Autodesk Inventor part; units mm, degrees
(part 3 of 7)
  line L373 (-46.0236, -59.4146) -> (-46.4209, -59.4428)
  line L374 (-46.4209, -59.4428) -> (-47.351, -59.469)
  line L375 (-47.351, -59.469) -> (-48.2632, -59.4537)
  line L376 (-48.2632, -59.4537) -> (-48.6381, -59.4301)
  line L377 (-48.6381, -59.4301) -> (-48.9193, -59.3956)
  line L378 (-48.9193, -59.3956) -> (-49.5759, -59.2467)
  line L379 (-49.5759, -59.2467) -> (-49.8747, -59.1544)
  line L380 (-49.8747, -59.1544) -> (-50.1547, -59.0499)
  line L381 (-50.1547, -59.0499) -> (-50.4164, -58.9329)
  line L382 (-50.4164, -58.9329) -> (-50.6606, -58.8031)
  line L383 (-50.6606, -58.8031) -> (-50.8877, -58.6602)
  line L384 (-50.8877, -58.6602) -> (-51.0986, -58.5041)
  line L385 (-51.0986, -58.5041) -> (-51.2624, -58.3746)
  line L386 (-51.2624, -58.3746) -> (-51.2624, -58.5384)
  line L387 (-51.2624, -58.5384) -> (-51.2496, -58.7821)
  line L388 (-51.2496, -58.7821) -> (-51.2138, -59.0766)
  line L389 (-51.2138, -59.0766) -> (-51.091, -59.7004)
  line L390 (-51.091, -59.7004) -> (-51.0286, -59.9871)
  line L391 (-51.0286, -59.9871) -> (-51.024, -60.0626)
  line L392 (-51.024, -60.0626) -> (-51.0376, -60.0967)
  line L393 (-51.0376, -60.0967) -> (-51.1136, -60.1071)
  line L394 (-51.1136, -60.1071) -> (-51.2372, -60.0829)
  line L395 (-51.2372, -60.0829) -> (-51.3971, -60.0265)
  line L396 (-51.3971, -60.0265) -> (-51.5825, -59.9405)
  line L397 (-51.5825, -59.9405) -> (-51.8754, -59.7765)
  line L398 (-51.8754, -59.7765) -> (-52.1087, -59.6085)
  line L399 (-52.1087, -59.6085) -> (-52.317, -59.4084)
  line L400 (-52.317, -59.4084) -> (-52.535, -59.148)
  line L401 (-52.535, -59.148) -> (-52.8359, -58.7594)
  line L402 (-52.8359, -58.7594) -> (-52.9541, -58.8318)
  line L403 (-52.9541, -58.8318) -> (-53.2253, -58.9829)
  line L404 (-53.2253, -58.9829) -> (-53.5098, -59.1066)
  line L405 (-53.5098, -59.1066) -> (-53.8365, -59.2138)
  line L406 (-53.8365, -59.2138) -> (-54.2342, -59.3156)
  line L407 (-54.2342, -59.3156) -> (-54.5443, -59.3742)
  line L408 (-54.5443, -59.3742) -> (-54.6227, -59.3762)
  line L409 (-54.6227, -59.3762) -> (-54.6571, -59.3614)
  line L410 (-54.6571, -59.3614) -> (-54.7009, -59.1688)
  line L411 (-54.7009, -59.1688) -> (-54.7357, -58.8151)
  line L412 (-54.7357, -58.8151) -> (-54.7541, -58.4136)
  line L413 (-54.7541, -58.4136) -> (-54.7486, -58.0774)
  line L414 (-54.7486, -58.0774) -> (-54.7195, -57.6626)
  line L415 (-54.7195, -57.6626) -> (-54.7329, -57.3906)
  line L416 (-54.7329, -57.3906) -> (-54.8113, -57.1344)
  line L417 (-54.8113, -57.1344) -> (-54.9772, -56.7667)
  line L418 (-54.9772, -56.7667) -> (-55.2401, -56.2067)
  line L419 (-55.2401, -56.2067) -> (-55.3772, -56.2067)
  line L420 (-55.3772, -56.2067) -> (-55.5187, -56.1843)
  line L421 (-55.5187, -56.1843) -> (-55.6744, -56.1305)
  line L422 (-55.6744, -56.1305) -> (-55.8426, -56.0168)
  line L423 (-55.8426, -56.0168) -> (-56.0768, -55.8128)
  line L424 (-56.0768, -55.8128) -> (-56.3318, -55.5609)
  line L425 (-56.3318, -55.5609) -> (-56.5621, -55.3037)
  line L426 (-56.5621, -55.3037) -> (-56.6955, -55.1437)
  line L427 (-56.6955, -55.1437) -> (-56.8631, -55.2999)
  line L428 (-56.8631, -55.2999) -> (-57.2147, -55.6065)
  line L429 (-57.2147, -55.6065) -> (-57.4899, -55.8214)
  line L430 (-57.4899, -55.8214) -> (-57.685, -55.9412)
  line L431 (-57.685, -55.9412) -> (-57.7515, -55.9645)
  line L432 (-57.7515, -55.9645) -> (-57.7966, -55.9628)
  line L433 (-57.7966, -55.9628) -> (-57.8301, -55.9383)
  line L434 (-57.8301, -55.9383) -> (-57.859, -55.8916)
  line L435 (-57.859, -55.8916) -> (-57.9018, -55.739)
  line L436 (-57.9018, -55.739) -> (-57.9225, -55.5192)
  line L437 (-57.9225, -55.5192) -> (-57.9185, -55.2466)
  line L438 (-57.9185, -55.2466) -> (-57.8994, -54.8808)
  line L439 (-57.8994, -54.8808) -> (-58.1128, -54.976)
  line L440 (-58.1128, -54.976) -> (-58.4276, -55.0851)
  line L441 (-58.4276, -55.0851) -> (-58.8824, -55.2199)
  line L442 (-58.8824, -55.2199) -> (-59.4996, -55.3913)
  line L443 (-59.4996, -55.3913) -> (-59.5345, -55.3951)
  line L444 (-59.5345, -55.3951) -> (-59.5554, -55.3789)
  line L445 (-59.5554, -55.3789) -> (-59.5682, -55.258)
  line L446 (-59.5682, -55.258) -> (-59.5539, -55.1342)
  line L447 (-59.5539, -55.1342) -> (-59.5329, -55.109)
  line L448 (-59.5329, -55.109) -> (-59.4996, -55.1018)
  line L449 (-59.4996, -55.1018) -> (-59.2636, -55.053)
  line L450 (-59.2636, -55.053) -> (-58.8515, -54.937)
  line L451 (-58.8515, -54.937) -> (-58.4158, -54.7996)
  line L452 (-58.4158, -54.7996) -> (-58.109, -54.6865)
  line L453 (-58.109, -54.6865) -> (-57.8376, -54.5834)
  line L454 (-57.8376, -54.5834) -> (-57.7515, -54.5766)
  line L455 (-57.7515, -54.5766) -> (-57.6927, -54.605)
  line L456 (-57.6927, -54.605) -> (-57.6572, -54.673)
  line L457 (-57.6572, -54.673) -> (-57.6407, -54.7845)
  line L458 (-57.6407, -54.7845) -> (-57.648, -55.1551)
  line L459 (-57.648, -55.1551) -> (-57.6585, -55.479)
  line L460 (-57.6585, -55.479) -> (-57.6404, -55.5971)
  line L461 (-57.6404, -55.5971) -> (-57.5546, -55.5456)
  line L462 (-57.5546, -55.5456) -> (-57.3856, -55.4085)
  line L463 (-57.3856, -55.4085) -> (-56.9165, -54.9799)
  line L464 (-56.9165, -54.9799) -> (-56.6841, -54.7551)
  line L465 (-56.6841, -54.7551) -> (-56.444, -55.0332)
  line L466 (-56.444, -55.0332) -> (-55.9573, -55.5656)
  line L467 (-55.9573, -55.5656) -> (-55.7882, -55.7233)
  line L468 (-55.7882, -55.7233) -> (-55.6477, -55.8295)
  line L469 (-55.6477, -55.8295) -> (-55.514, -55.9035)
  line L470 (-55.514, -55.9035) -> (-55.4153, -55.9362)
  line L471 (-55.4153, -55.9362) -> (-55.3595, -55.9259)
  line L472 (-55.3595, -55.9259) -> (-55.3544, -55.8714)
  line L473 (-55.3544, -55.8714) -> (-55.4462, -55.5283)
  line L474 (-55.4462, -55.5283) -> (-55.5234, -55.1751)
  line L475 (-55.5234, -55.1751) -> (-55.6439, -54.3817)
  line L476 (-55.6439, -54.3817) -> (-55.6632, -54.1753)
  line L477 (-55.6632, -54.1753) -> (-55.6525, -54.0593)
  line L478 (-55.6525, -54.0593) -> (-55.6332, -54.0272)
  line L479 (-55.6332, -54.0272) -> (-55.6032, -54.0082)
  line L480 (-55.6032, -54.0082) -> (-55.5068, -53.9969)
  line L481 (-55.5068, -53.9969) -> (-55.4609, -54.0075)
  line L482 (-55.4609, -54.0075) -> (-55.431, -54.0559)
  line L483 (-55.431, -54.0559) -> (-55.381, -54.3664)
  line L484 (-55.381, -54.3664) -> (-55.2779, -55.0469)
  line L485 (-55.2779, -55.0469) -> (-55.142, -55.6209)
  line L486 (-55.142, -55.6209) -> (-54.9417, -56.1935)
  line L487 (-54.9417, -56.1935) -> (-54.6457, -56.8696)
  line L488 (-54.6457, -56.8696) -> (-54.5187, -57.1502)
  line L489 (-54.5187, -57.1502) -> (-54.4528, -57.3254)
  line L490 (-54.4528, -57.3254) -> (-54.4319, -57.4499)
  line L491 (-54.4319, -57.4499) -> (-54.44, -57.5783)
  line L492 (-54.44, -57.5783) -> (-54.4923, -58.2436)
  line L493 (-54.4923, -58.2436) -> (-54.4819, -58.7403)
  line L494 (-54.4819, -58.7403) -> (-54.4552, -59.0718)
  line L495 (-54.4552, -59.0718) -> (-54.2723, -59.0489)
  line L496 (-54.2723, -59.0489) -> (-54.006, -58.9912)
  line L497 (-54.006, -58.9912) -> (-53.6994, -58.8899)
  line L498 (-53.6994, -58.8899) -> (-53.3877, -58.7585)
  line L499 (-53.3877, -58.7585) -> (-53.1065, -58.6108)
  line L500 (-53.1065, -58.6108) -> (-52.7674, -58.4165)
  line L501 (-52.7674, -58.4165) -> (-52.5197, -58.7441)
  line L502 (-52.5197, -58.7441) -> (-52.2934, -59.0362)
  line L503 (-52.2934, -59.0362) -> (-52.0778, -59.2718)
  line L504 (-52.0778, -59.2718) -> (-51.865, -59.4589)
  line L505 (-51.865, -59.4589) -> (-51.6472, -59.6052)
  line L506 (-51.6472, -59.6052) -> (-51.3881, -59.7347)
  line L507 (-51.3881, -59.7347) -> (-51.4339, -59.3842)
  line L508 (-51.4339, -59.3842) -> (-51.4843, -58.9908)
  line L509 (-51.4843, -58.9908) -> (-51.5177, -58.5232)
  line L510 (-51.5177, -58.5232) -> (-51.5258, -58.0845)
  line L511 (-51.5258, -58.0845) -> (-51.5107, -58.0051)
  line L512 (-51.5107, -58.0051) -> (-51.4796, -57.9745)
  line L513 (-51.4796, -57.9745) -> (-51.4248, -57.9843)
  line L514 (-51.4248, -57.9843) -> (-51.3243, -58.0355)
  line L515 (-51.3243, -58.0355) -> (-50.9919, -58.2565)
  line L516 (-50.9919, -58.2565) -> (-50.6288, -58.4993)
  line L517 (-50.6288, -58.4993) -> (-50.279, -58.6988)
  line L518 (-50.279, -58.6988) -> (-49.9286, -58.859)
  line L519 (-49.9286, -58.859) -> (-49.5636, -58.9837)
  line L520 (-49.5636, -58.9837) -> (-49.1703, -59.0768)
  line L521 (-49.1703, -59.0768) -> (-48.7347, -59.1421)
  line L522 (-48.7347, -59.1421) -> (-48.2429, -59.1836)
  line L523 (-48.2429, -59.1836) -> (-47.681, -59.2051)
  line L524 (-47.681, -59.2051) -> (-47.0912, -59.2088)
  line L525 (-47.0912, -59.2088) -> (-46.5442, -59.1902)
  line L526 (-46.5442, -59.1902) -> (-46.0308, -59.1477)
  line L527 (-46.0308, -59.1477) -> (-45.5417, -59.0799)
  line L528 (-45.5417, -59.0799) -> (-45.0676, -58.9851)
  line L529 (-45.0676, -58.9851) -> (-44.5992, -58.8617)
  line L530 (-44.5992, -58.8617) -> (-44.1272, -58.7083)
  line L531 (-44.1272, -58.7083) -> (-43.6424, -58.5232)
  line L532 (-43.6424, -58.5232) -> (-42.8547, -58.1674)
  line L533 (-42.8547, -58.1674) -> (-42.4969, -57.9922)
  line L534 (-42.4969, -57.9922) -> (-42.347, -57.9059)
  line L535 (-42.347, -57.9059) -> (-42.8047, -57.504)
  line L536 (-42.8047, -57.504) -> (-43.5853, -56.8734)
  line L537 (-43.5853, -56.8734) -> (-44.1782, -56.421)
  line L538 (-44.1782, -56.421) -> (-44.9912, -55.8257)
  line L539 (-44.9912, -55.8257) -> (-46.1875, -54.9379)
  line L540 (-46.1875, -54.9379) -> (-46.503, -54.6984)
  line L541 (-46.503, -54.6984) -> (-46.6742, -54.5822)
  line L542 (-46.6742, -54.5822) -> (-46.7554, -54.5581)
  line L543 (-46.7554, -54.5581) -> (-46.8009, -54.595)
  line L544 (-46.8009, -54.595) -> (-47.0181, -54.8808)
  line L545 (-47.0181, -54.8808) -> (-47.1397, -55.0219)
  line L546 (-47.1397, -55.0219) -> (-47.251, -55.118)
  line L547 (-47.251, -55.118) -> (-47.3487, -55.1669)
  line L548 (-47.3487, -55.1669) -> (-47.4296, -55.1665)
  line L549 (-47.4296, -55.1665) -> (-47.4824, -55.1084)
  line L550 (-47.4824, -55.1084) -> (-47.5324, -54.9989)
  line L551 (-47.5324, -54.9989) -> (-47.5697, -54.7039)
  line L552 (-47.5697, -54.7039) -> (-47.5934, -54.1902)
  line L553 (-47.5934, -54.1902) -> (-47.5999, -53.6037)
  line L554 (-47.5999, -53.6037) -> (-47.5858, -53.0901)
  line L555 (-47.5858, -53.0901) -> (-47.5591, -52.6634)
  line L556 (-47.5591, -52.6634) -> (-47.4334, -52.6634)
  line L557 (-47.4334, -52.6634) -> (-47.3076, -52.6634)
  line L558 (-47.3076, -52.6634) -> (-47.3267, -53.6425)
  line L559 (-47.3267, -53.6425) -> (-47.3305, -54.3712)
  line L560 (-47.3305, -54.3712) -> (-47.3114, -54.717)
  line L561 (-47.3114, -54.717) -> (-47.2852, -54.7565)
  line L562 (-47.2852, -54.7565) -> (-47.2443, -54.7365)
  line L563 (-47.2443, -54.7365) -> (-47.0371, -54.4388)
  line L564 (-47.0371, -54.4388) -> (-46.8209, -54.0755)
  line L565 (-46.8209, -54.0755) -> (-46.6333, -53.7149)
  line L566 (-46.6333, -53.7149) -> (-46.4656, -53.3568)
  line L567 (-46.4656, -53.3568) -> (-46.138, -53.5282)
  line L568 (-46.138, -53.5282) -> (-45.841, -53.673)
  line L569 (-45.841, -53.673) -> (-45.5822, -53.7749)
  line L570 (-45.5822, -53.7749) -> (-45.3413, -53.8411)
  line L571 (-45.3413, -53.8411) -> (-45.0978, -53.8788)
  line L572 (-45.0978, -53.8788) -> (-44.8235, -53.9054)
  line L573 (-44.8235, -53.9054) -> (-44.8235, -53.7492)
  line L574 (-44.8235, -53.7492) -> (-44.8364, -53.5208)
  line L575 (-44.8364, -53.5208) -> (-44.8697, -53.2392)
  line L576 (-44.8697, -53.2392) -> (-44.9645, -52.7434)
  line L577 (-44.9645, -52.7434) -> (-45.0376, -52.5217)
  line L578 (-45.0376, -52.5217) -> (-45.1318, -52.299)
  line L579 (-45.1318, -52.299) -> (-45.2477, -52.074)
  line L580 (-45.2477, -52.074) -> (-45.386, -51.8456)
  line L581 (-45.386, -51.8456) -> (-45.7323, -51.3745)
  line L582 (-45.7323, -51.3745) -> (-46.1761, -50.8765)
  line L583 (-46.1761, -50.8765) -> (-46.4613, -50.5689)
  line L584 (-46.4613, -50.5689) -> (-46.6152, -50.3678)
  line L585 (-46.6152, -50.3678) -> (-46.6486, -50.2972)
  line L586 (-46.6486, -50.2972) -> (-46.6561, -50.241)
  line L587 (-46.6561, -50.241) -> (-46.6401, -50.1955)
  line L588 (-46.6401, -50.1955) -> (-46.6028, -50.1564)
  line L589 (-46.6028, -50.1564) -> (-46.1761, -49.9583)
  line L590 (-46.1761, -49.9583) -> (-45.7307, -49.7577)
  line L591 (-45.7307, -49.7577) -> (-45.3236, -49.5492)
  line L592 (-45.3236, -49.5492) -> (-44.9464, -49.3265)
  line L593 (-44.9464, -49.3265) -> (-44.5911, -49.0834)
  line L594 (-44.5911, -49.0834) -> (-44.2493, -48.8137)
  line L595 (-44.2493, -48.8137) -> (-43.9129, -48.5111)
  line L596 (-43.9129, -48.5111) -> (-43.5737, -48.1696)
  line L597 (-43.5737, -48.1696) -> (-43.2233, -47.7828)
  line L598 (-43.2233, -47.7828) -> (-42.8931, -47.3882)
  line L599 (-42.8931, -47.3882) -> (-42.5847, -46.9922)
  line L600 (-42.5847, -46.9922) -> (-42.3612, -46.679)
  line L601 (-42.3612, -46.679) -> (-42.3012, -46.5799)
  line L602 (-42.3012, -46.5799) -> (-42.2861, -46.5331)
  line L603 (-42.2861, -46.5331) -> (-42.4023, -46.4588)
  line L604 (-42.4023, -46.4588) -> (-42.6442, -46.3388)
  line L605 (-42.6442, -46.3388) -> (-43.1841, -46.1064)
  line L606 (-43.1841, -46.1064) -> (-43.7177, -45.923)
  line L607 (-43.7177, -45.923) -> (-44.2783, -45.7789)
  line L608 (-44.2783, -45.7789) -> (-44.8997, -45.6644)
  line L609 (-44.8997, -45.6644) -> (-45.1951, -45.6319)
  line L610 (-45.1951, -45.6319) -> (-45.584, -45.6087)
  line L611 (-45.584, -45.6087) -> (-46.5218, -45.5901)
  line L612 (-46.5218, -45.5901) -> (-47.4725, -45.6087)
  line L613 (-47.4725, -45.6087) -> (-47.8775, -45.6319)
  line L614 (-47.8775, -45.6319) -> (-48.1954, -45.6644)
  line L615 (-48.1954, -45.6644) -> (-48.6777, -45.7431)
  line L616 (-48.6777, -45.7431) -> (-49.0923, -45.8345)
  line L617 (-49.0923, -45.8345) -> (-49.4508, -45.9445)
  line L618 (-49.4508, -45.9445) -> (-49.7646, -46.0792)
  line L619 (-49.7646, -46.0792) -> (-50.0454, -46.2444)
  line L620 (-50.0454, -46.2444) -> (-50.3047, -46.4461)
  line L621 (-50.3047, -46.4461) -> (-50.5542, -46.6902)
  line L622 (-50.5542, -46.6902) -> (-50.8052, -46.9827)
  line L623 (-50.8052, -46.9827) -> (-51.0529, -47.2913)
  line L624 (-51.0529, -47.2913) -> (-51.0719, -46.495)
  line L625 (-51.0719, -46.495) -> (-51.0929, -45.9254)
  line L626 (-51.0929, -45.9254) -> (-51.1138, -45.6758)
  line L627 (-51.1138, -45.6758) -> (-51.1663, -45.682)
  line L628 (-51.1663, -45.682) -> (-51.2692, -45.7464)
  line L629 (-51.2692, -45.7464) -> (-51.591, -46.0178)
  line L630 (-51.591, -46.0178) -> (-52.0086, -46.4248)
  line L631 (-52.0086, -46.4248) -> (-52.4511, -46.9026)
  line L632 (-52.4511, -46.9026) -> (-52.6302, -47.1046)
  line L633 (-52.6302, -47.1046) -> (-53.0036, -46.8112)
  line L634 (-53.0036, -46.8112) -> (-53.3412, -46.5575)
  line L635 (-53.3412, -46.5575) -> (-53.6846, -46.3188)
  line L636 (-53.6846, -46.3188) -> (-53.9637, -46.1415)
  line L637 (-53.9637, -46.1415) -> (-54.1085, -46.0721)
  line L638 (-54.1085, -46.0721) -> (-54.1472, -46.101)
  line L639 (-54.1472, -46.101) -> (-54.1866, -46.1978)
  line L640 (-54.1866, -46.1978) -> (-54.2876, -46.655)
  line L641 (-54.2876, -46.655) -> (-54.3471, -47.0104)
  line L642 (-54.3471, -47.0104) -> (-54.3728, -47.3094)
  line L643 (-54.3728, -47.3094) -> (-54.3663, -47.584)
  line L644 (-54.3663, -47.584) -> (-54.3295, -47.8666)
  line L645 (-54.3295, -47.8666) -> (-54.2685, -48.2361)
  line L646 (-54.2685, -48.2361) -> (-54.4971, -48.6857)
  line L647 (-54.4971, -48.6857) -> (-54.7133, -49.1758)
  line L648 (-54.7133, -49.1758) -> (-54.9124, -49.7144)
  line L649 (-54.9124, -49.7144) -> (-55.1372, -50.3545)
  line L650 (-55.1372, -50.3545) -> (-55.1605, -50.3793)
  line L651 (-55.1605, -50.3793) -> (-55.1977, -50.3755)
  line L652 (-55.1977, -50.3755) -> (-55.3582, -50.2593)
  line L653 (-55.3582, -50.2593) -> (-55.7522, -49.9425)
  line L654 (-55.7522, -49.9425) -> (-56.1258, -49.6651)
  line L655 (-56.1258, -49.6651) -> (-56.4836, -49.4243)
  line L656 (-56.4836, -49.4243) -> (-56.8303, -49.2177)
  line L657 (-56.8303, -49.2177) -> (-57.1703, -49.0427)
  line L658 (-57.1703, -49.0427) -> (-57.5083, -48.8968)
  line L659 (-57.5083, -48.8968) -> (-57.8488, -48.7774)
  line L660 (-57.8488, -48.7774) -> (-58.1966, -48.6819)
  line L661 (-58.1966, -48.6819) -> (-58.9077, -48.5614)
  line L662 (-58.9077, -48.5614) -> (-59.553, -48.4724)
  line L663 (-59.553, -48.4724) -> (-59.5682, -48.339)
  line L664 (-59.5682, -48.339) -> (-59.5657, -48.2616)
  line L665 (-59.5657, -48.2616) -> (-59.5511, -48.2228)
  line L666 (-59.5511, -48.2228) -> (-59.5136, -48.2126)
  line L667 (-59.5136, -48.2126) -> (-59.4425, -48.2209)
  line L668 (-59.4425, -48.2209) -> (-58.9586, -48.2819)
  line L669 (-58.9586, -48.2819) -> (-58.5007, -48.3508)
  line L670 (-58.5007, -48.3508) -> (-58.0528, -48.452)
  line L671 (-58.0528, -48.452) -> (-57.6149, -48.5855)
  line L672 (-57.6149, -48.5855) -> (-57.187, -48.7514)
  line L673 (-57.187, -48.7514) -> (-56.7691, -48.9499)
  line L674 (-56.7691, -48.9499) -> (-56.3612, -49.1809)
  line L675 (-56.3612, -49.1809) -> (-55.9632, -49.4446)
  line L676 (-55.9632, -49.4446) -> (-55.5753, -49.7411)
  line L677 (-55.5753, -49.7411) -> (-55.2858, -49.9545)
  line L678 (-55.2858, -49.9545) -> (-55.1105, -49.463)
  line L679 (-55.1105, -49.463) -> (-54.9376, -49.0091)
  line L680 (-54.9376, -49.0091) -> (-54.7448, -48.5867)
  line L681 (-54.7448, -48.5867) -> (-54.5352, -48.1904)
  line L682 (-54.5352, -48.1904) -> (-54.5847, -47.9771)
  line L683 (-54.5847, -47.9771) -> (-54.6192, -47.7031)
  line L684 (-54.6192, -47.7031) -> (-54.6262, -47.3598)
  line L685 (-54.6262, -47.3598) -> (-54.6067, -46.9966)
  line L686 (-54.6067, -46.9966) -> (-54.5619, -46.6626)
  line L687 (-54.5619, -46.6626) -> (-54.4295, -46.0783)
  line L688 (-54.4295, -46.0783) -> (-54.3142, -45.7025)
  line L689 (-54.3142, -45.7025) -> (-54.2724, -45.6989)
  line L690 (-54.2724, -45.6989) -> (-54.1791, -45.733)
  line L691 (-54.1791, -45.733) -> (-53.8761, -45.8925)
  line L692 (-53.8761, -45.8925) -> (-53.4816, -46.137)
  line L693 (-53.4816, -46.137) -> (-53.0722, -46.4226)
  line L694 (-53.0722, -46.4226) -> (-52.6683, -46.7236)
  line L695 (-52.6683, -46.7236) -> (-52.1273, -46.1749)
  line L696 (-52.1273, -46.1749) -> (-51.6787, -45.7454)
  line L697 (-51.6787, -45.7454) -> (-51.3615, -45.4815)
  line L698 (-51.3615, -45.4815) -> (-51.1965, -45.3911)
  line L699 (-51.1965, -45.3911) -> (-51.0557, -45.3439)
  line L700 (-51.0557, -45.3439) -> (-50.9479, -45.3417)
  line L701 (-50.9479, -45.3417) -> (-50.9089, -45.358)
  line L702 (-50.9089, -45.358) -> (-50.8814, -45.3863)
  line L703 (-50.8814, -45.3863) -> (-50.849, -45.5564)
  line L704 (-50.849, -45.5564) -> (-50.8247, -45.873)
  line L705 (-50.8247, -45.873) -> (-50.8155, -46.2082)
  line L706 (-50.8155, -46.2082) -> (-50.8281, -46.434)
  line L707 (-50.8281, -46.434) -> (-50.8547, -46.5864)
  line L708 (-50.8547, -46.5864) -> (-50.588, -46.3388)
  line L709 (-50.588, -46.3388) -> (-50.3729, -46.1542)
  line L710 (-50.3729, -46.1542) -> (-50.1464, -45.9935)
  line L711 (-50.1464, -45.9935) -> (-49.9026, -45.8542)
  line L712 (-49.9026, -45.8542) -> (-49.6355, -45.7339)
  line L713 (-49.6355, -45.7339) -> (-49.3392, -45.6305)
  line L714 (-49.3392, -45.6305) -> (-49.0075, -45.5415)
  line L715 (-49.0075, -45.5415) -> (-48.6346, -45.4647)
  line L716 (-48.6346, -45.4647) -> (-48.2144, -45.3977)
  line L717 (-48.2144, -45.3977) -> (-47.9027, -45.3664)
  line L718 (-47.9027, -45.3664) -> (-47.502, -45.3441)
  line L719 (-47.502, -45.3441) -> (-46.5528, -45.3263)
  line L720 (-46.5528, -45.3263) -> (-45.6057, -45.3441)
  line L721 (-45.6057, -45.3441) -> (-45.2076, -45.3664)
  line L722 (-45.2076, -45.3664) -> (-44.8997, -45.3977)
  line L723 (-44.8997, -45.3977) -> (-44.4631, -45.4716)
  line L724 (-44.4631, -45.4716) -> (-44.0186, -45.5687)
  line L725 (-44.0186, -45.5687) -> (-43.5956, -45.6822)
  line L726 (-43.5956, -45.6822) -> (-43.2233, -45.8054)
  line L727 (-43.2233, -45.8054) -> (-42.8685, -45.9513)
  line L728 (-42.8685, -45.9513) -> (-42.4308, -46.1502)
  line L729 (-42.4308, -46.1502) -> (-42.0532, -46.3347)
  line L730 (-42.0532, -46.3347) -> (-41.8784, -46.4378)
  line L731 (-41.8784, -46.4378) -> (-41.966, -46.5964)
  line L732 (-41.966, -46.5964) -> (-42.2022, -46.9293)
  line L733 (-49.7651, -50.3088) -> (-49.7765, -51.4442)
  line L734 (-49.7765, -51.4442) -> (-50.6261, -51.4442)
  line L735 (-50.6261, -51.4442) -> (-51.6167, -51.4213)
  line L736 (-51.6167, -51.4213) -> (-51.8051, -51.3628)
  line L737 (-51.8051, -51.3628) -> (-51.9863, -51.2589)
  line L738 (-51.9863, -51.2589) -> (-52.1418, -51.1229)
  line L739 (-52.1418, -51.1229) -> (-52.253, -50.9679)
  line L740 (-52.253, -50.9679) -> (-52.3123, -50.8206)
  line L741 (-52.3123, -50.8206) -> (-52.3452, -50.6654)
  line L742 (-52.3452, -50.6654) -> (-52.3527, -50.508)
  line L743 (-52.3527, -50.508) -> (-52.3359, -50.354)
  line L744 (-52.3359, -50.354) -> (-52.2959, -50.2092)
  line L745 (-52.2959, -50.2092) -> (-52.2337, -50.0791)
  line L746 (-52.2337, -50.0791) -> (-52.1505, -49.9694)
  line L747 (-52.1505, -49.9694) -> (-52.0473, -49.8859)
  line L748 (-52.0473, -49.8859) -> (-51.8394, -49.7791)
  line L749 (-51.8394, -49.7791) -> (-51.5986, -49.7149)
  line L750 (-51.5986, -49.7149) -> (-51.265, -49.6828)
  line L751 (-51.265, -49.6828) -> (-50.7785, -49.6725)
  line L752 (-50.7785, -49.6725) -> (-50.047, -49.6725)
  line L753 (-50.047, -49.6725) -> (-50.0242, -49.4439)
  line L754 (-50.0242, -49.4439) -> (-50.0099, -49.2277)
  line L755 (-50.0099, -49.2277) -> (-50.0127, -49.0286)
  line L756 (-50.0127, -49.0286) -> (-50.0226, -48.9228)
  line L757 (-50.0226, -48.9228) -> (-50.0461, -48.8596)
  line L758 (-50.0461, -48.8596) -> (-50.0995, -48.817)
  line L759 (-50.0995, -48.817) -> (-50.1994, -48.7734)
  line L760 (-50.1994, -48.7734) -> (-50.3992, -48.7092)
  line L761 (-50.3992, -48.7092) -> (-50.6307, -48.6573)
  line L762 (-50.6307, -48.6573) -> (-51.1438, -48.5933)
  line L763 (-51.1438, -48.5933) -> (-51.6476, -48.588)
  line L764 (-51.6476, -48.588) -> (-51.8676, -48.6093)
  line L765 (-51.8676, -48.6093) -> (-52.0511, -48.6476)
  line L766 (-52.0511, -48.6476) -> (-52.2021, -48.6862)
  line L767 (-52.2021, -48.6862) -> (-52.2759, -48.6933)
  line L768 (-52.2759, -48.6933) -> (-52.314, -48.56)
  line L769 (-52.314, -48.56) -> (-52.3368, -48.4457)
  line L770 (-52.3368, -48.4457) -> (-52.0625, -48.3771)
  line L771 (-52.0625, -48.3771) -> (-51.9041, -48.3453)
  line L772 (-51.9041, -48.3453) -> (-51.7382, -48.3285)
  line L773 (-51.7382, -48.3285) -> (-51.251, -48.3314)
  line L774 (-51.251, -48.3314) -> (-50.9231, -48.35)
  line L775 (-50.9231, -48.35) -> (-50.6542, -48.3833)
  line L776 (-50.6542, -48.3833) -> (-50.3932, -48.4402)
  line L777 (-50.3932, -48.4402) -> (-50.0889, -48.5295)
  line L778 (-50.0889, -48.5295) -> (-50.0405, -48.5396)
  line L779 (-50.0405, -48.5396) -> (-50.0156, -48.5128)
  line L780 (-50.0156, -48.5128) -> (-50.0051, -48.2476)
  line L781 (-50.0051, -48.2476) -> (-50.0051, -47.939)
  line L782 (-50.0051, -47.939) -> (-49.8718, -47.939)
  line L783 (-49.8718, -47.939) -> (-49.7384, -47.939)
  line L784 (-49.7384, -47.939) -> (-49.746, -48.5562)
  line L785 (-49.746, -48.5562) -> (-49.7651, -50.3088)
  line L786 (-49.8794, -56.6524) -> (-49.8908, -57.5021)
  line L787 (-49.8908, -57.5021) -> (-50.0242, -57.5021)
  line L788 (-50.0242, -57.5021) -> (-50.1575, -57.5021)
  line L789 (-50.1575, -57.5021) -> (-50.1575, -57.2163)
  line L790 (-50.1575, -57.2163) -> (-50.1575, -56.9306)
  line L791 (-50.1575, -56.9306) -> (-50.3099, -57.0068)
  line L792 (-50.3099, -57.0068) -> (-50.5067, -57.0864)
  line L793 (-50.5067, -57.0864) -> (-50.7414, -57.1463)
  line L794 (-50.7414, -57.1463) -> (-51.0032, -57.1841)
  line L795 (-51.0032, -57.1841) -> (-51.2815, -57.1973)
  line L796 (-51.2815, -57.1973) -> (-51.5308, -57.19)
  line L797 (-51.5308, -57.19) -> (-51.7449, -57.1644)
  line L798 (-51.7449, -57.1644) -> (-51.9539, -57.1153)
  line L799 (-51.9539, -57.1153) -> (-52.1882, -57.0373)
  line L800 (-52.1882, -57.0373) -> (-52.3654, -56.9572)
  line L801 (-52.3654, -56.9572) -> (-52.3886, -56.9215)
  line L802 (-52.3886, -56.9215) -> (-52.3826, -56.8772)
  line L803 (-52.3826, -56.8772) -> (-52.3479, -56.7967)
  line L804 (-52.3479, -56.7967) -> (-52.2883, -56.7648)
  line L805 (-52.2883, -56.7648) -> (-52.1757, -56.7786)
  line L806 (-52.1757, -56.7786) -> (-51.9825, -56.8353)
  line L807 (-51.9825, -56.8353) -> (-51.6891, -56.912)
  line L808 (-51.6891, -56.912) -> (-51.4301, -56.9572)
  line L809 (-51.4301, -56.9572) -> (-51.1761, -56.955)
  line L810 (-51.1761, -56.955) -> (-50.8843, -56.9139)
  line L811 (-50.8843, -56.9139) -> (-50.5996, -56.842)
  line L812 (-50.5996, -56.842) -> (-50.3671, -56.7477)
  line L813 (-50.3671, -56.7477) -> (-50.1766, -56.6448)
  line L814 (-50.1766, -56.6448) -> (-50.1461, -56.2105)
  line L815 (-50.1461, -56.2105) -> (-50.1308, -55.7342)
  line L816 (-50.1308, -55.7342) -> (-50.1598, -55.7164)
  line L817 (-50.1598, -55.7164) -> (-50.2337, -55.709)
  line L818 (-50.2337, -55.709) -> (-50.5423, -55.7266)
  line L819 (-50.5423, -55.7266) -> (-50.8343, -55.7427)
  line L820 (-50.8343, -55.7427) -> (-51.1132, -55.7372)
  line L821 (-51.1132, -55.7372) -> (-51.3748, -55.7112)
  line L822 (-51.3748, -55.7112) -> (-51.6148, -55.6657)
  line L823 (-51.6148, -55.6657) -> (-51.8292, -55.6015)
  line L824 (-51.8292, -55.6015) -> (-52.0136, -55.5198)
  line L825 (-52.0136, -55.5198) -> (-52.1639, -55.4215)
  line L826 (-52.1639, -55.4215) -> (-52.2759, -55.3075)
  line L827 (-52.2759, -55.3075) -> (-52.3349, -55.2219)
  line L828 (-52.3349, -55.2219) -> (-52.3683, -55.1399)
  line L829 (-52.3683, -55.1399) -> (-52.383, -55.0321)
  line L830 (-52.383, -55.0321) -> (-52.3864, -54.8694)
  line L831 (-52.3864, -54.8694) -> (-52.3707, -54.6103)
  line L832 (-52.3707, -54.6103) -> (-52.3462, -54.5318)
  line L833 (-52.3462, -54.5318) -> (-52.3064, -54.4655)
  line L834 (-52.3064, -54.4655) -> (-52.2055, -54.3531)
  line L835 (-52.2055, -54.3531) -> (-52.0816, -54.2605)
  line L836 (-52.0816, -54.2605) -> (-51.9286, -54.1863)
  line L837 (-51.9286, -54.1863) -> (-51.7401, -54.1288)
  line L838 (-51.7401, -54.1288) -> (-51.51, -54.0865)
  line L839 (-51.51, -54.0865) -> (-51.2321, -54.0578)
  line L840 (-51.2321, -54.0578) -> (-50.508, -54.035)
  line L841 (-50.508, -54.035) -> (-49.8527, -54.035)
  line L842 (-49.8527, -54.035) -> (-49.8603, -54.9189)
  line L843 (-49.8603, -54.9189) -> (-49.8794, -56.6524)
  line L844 (-52.4702, -53.3034) -> (-52.4824, -53.3711)
  line L845 (-52.4824, -53.3711) -> (-52.5021, -53.4077)
  line L846 (-52.5021, -53.4077) -> (-52.5382, -53.4208)
  line L847 (-52.5382, -53.4208) -> (-52.5997, -53.4178)
  line L848 (-52.5997, -53.4178) -> (-52.714, -53.4063)
  line L849 (-52.714, -53.4063) -> (-52.7255, -52.9796)
  line L850 (-52.7255, -52.9796) -> (-52.7407, -52.5567)
  line L851 (-52.7407, -52.5567) -> (-52.6378, -52.5376)
  line L852 (-52.6378, -52.5376) -> (-52.5612, -52.531)
  line L853 (-52.5612, -52.531) -> (-52.5159, -52.5414)
  line L854 (-52.5159, -52.5414) -> (-52.4916, -52.6525)
  line L855 (-52.4916, -52.6525) -> (-52.473, -52.8753)
  line L856 (-52.473, -52.8753) -> (-52.4702, -53.3034)
  line L857 (-52.916, -48.4495) -> (-53.2017, -48.7391)
  line L858 (-53.2017, -48.7391) -> (-52.9769, -48.7391)
  line L859 (-52.9769, -48.7391) -> (-52.7883, -48.7538)
  line L860 (-52.7883, -48.7538) -> (-52.7422, -48.776)
  line L861 (-52.7422, -48.776) -> (-52.714, -48.8115)
  line L862 (-52.714, -48.8115) -> (-52.6997, -48.8562)
  line L863 (-52.6997, -48.8562) -> (-52.7112, -48.9124)
  line L864 (-52.7112, -48.9124) -> (-52.8283, -49.1048)
  line L865 (-52.8283, -49.1048) -> (-53.0607, -49.4515)
  line L866 (-53.0607, -49.4515) -> (-53.1144, -49.5344)
  line L867 (-53.1144, -49.5344) -> (-53.156, -49.5687)
  line L868 (-53.156, -49.5687) -> (-53.2033, -49.5587)
  line L869 (-53.2033, -49.5587) -> (-53.2741, -49.5087)
  line L870 (-53.2741, -49.5087) -> (-53.3617, -49.4401)
  line L871 (-53.3617, -49.4401) -> (-53.2055, -49.2267)
  line L872 (-53.2055, -49.2267) -> (-53.0531, -48.9905)
  line L873 (-53.0531, -48.9905) -> (-53.1126, -48.9748)
  line L874 (-53.1126, -48.9748) -> (-53.255, -48.9677)
  line L875 (-53.255, -48.9677) -> (-53.3909, -48.9586)
  line L876 (-53.3909, -48.9586) -> (-53.4817, -48.9296)
  line L877 (-53.4817, -48.9296) -> (-53.5326, -48.8777)
  line L878 (-53.5326, -48.8777) -> (-53.5484, -48.8)
  line L879 (-53.5484, -48.8) -> (-53.439, -48.6485)
  line L880 (-53.439, -48.6485) -> (-53.1931, -48.3819)
  line L881 (-53.1931, -48.3819) -> (-52.9344, -48.1282)
  line L882 (-52.9344, -48.1282) -> (-52.7864, -48.0152)
  line L883 (-52.7864, -48.0152) -> (-52.695, -48.0876)
  line L884 (-52.695, -48.0876) -> (-52.6636, -48.1339)
  line L885 (-52.6636, -48.1339) -> (-52.6783, -48.19)
  line L886 (-52.6783, -48.19) -> (-52.916, -48.4495)
  line L887 (-52.7636, -57.3306) -> (-52.8817, -57.6164)
  line L888 (-52.8817, -57.6164) -> (-53.0803, -57.924)
  line L889 (-53.0803, -57.924) -> (-53.1855, -58.0568)
  line L890 (-53.1855, -58.0568) -> (-53.2474, -58.1117)
  line L891 (-53.2474, -58.1117) -> (-53.3579, -58.0431)
  line L892 (-53.3579, -58.0431) -> (-53.4417, -57.9745)
  line L893 (-53.4417, -57.9745) -> (-53.3008, -57.8069)
  line L894 (-53.3008, -57.8069) -> (-53.1146, -57.5445)
  line L895 (-53.1146, -57.5445) -> (-53.0698, -57.4495)
  line L896 (-53.0698, -57.4495) -> (-53.0684, -57.3992)
  line L897 (-53.0684, -57.3992) -> (-53.146, -57.4011)
  line L898 (-53.146, -57.4011) -> (-53.3008, -57.4373)
  line L899 (-53.3008, -57.4373) -> (-53.4341, -57.4692)
  line L900 (-53.4341, -57.4692) -> (-53.5315, -57.4765)
  line L901 (-53.5315, -57.4765) -> (-53.5934, -57.4556)
  line L902 (-53.5934, -57.4556) -> (-53.6203, -57.4025)
  line L903 (-53.6203, -57.4025) -> (-53.6128, -57.3136)
  line L904 (-53.6128, -57.3136) -> (-53.5713, -57.1849)
  line L905 (-53.5713, -57.1849) -> (-53.3884, -56.7934)
  line L906 (-53.3884, -56.7934) -> (-53.1522, -56.3286)
  line L907 (-53.1522, -56.3286) -> (-53.0455, -56.3819)
  line L908 (-53.0455, -56.3819) -> (-52.9388, -56.4353)
  line L909 (-52.9388, -56.4353) -> (-53.1103, -56.7782)
  line L910 (-53.1103, -56.7782) -> (-53.2817, -57.1439)
  line L911 (-53.2817, -57.1439) -> (-53.1974, -57.152)
  line L912 (-53.1974, -57.152) -> (-52.996, -57.1401)
  line L913 (-52.996, -57.1401) -> (-52.795, -57.1311)
  line L914 (-52.795, -57.1311) -> (-52.714, -57.1477)
  line L915 (-52.714, -57.1477) -> (-52.7636, -57.3306)
  line L916 (-53.4875, -51.2727) -> (-53.5922, -51.3746)
  line L917 (-53.5922, -51.3746) -> (-53.6627, -51.4823)
  line L918 (-53.6627, -51.4823) -> (-53.6857, -51.5684)
  line L919 (-53.6857, -51.5684) -> (-53.6977, -51.6849)
  line L920 (-53.6977, -51.6849) -> (-53.6913, -51.98)
  line L921 (-53.6913, -51.98) -> (-53.6477, -52.3101)
  line L922 (-53.6477, -52.3101) -> (-53.5713, -52.6176)
  line L923 (-53.5713, -52.6176) -> (-53.4684, -52.9301)
  line L924 (-53.4684, -52.9301) -> (-53.636, -53.1701)
  line L925 (-53.636, -53.1701) -> (-53.8433, -53.4865)
  line L926 (-53.8433, -53.4865) -> (-53.907, -53.6119)
  line L927 (-53.907, -53.6119) -> (-53.9456, -53.7211)
  line L928 (-53.9456, -53.7211) -> (-53.9603, -53.8184)
  line L929 (-53.9603, -53.8184) -> (-53.9522, -53.9079)
  line L930 (-53.9522, -53.9079) -> (-53.9224, -53.9939)
  line L931 (-53.9224, -53.9939) -> (-53.8723, -54.0807)
  line L932 (-53.8723, -54.0807) -> (-53.777, -54.256)
  line L933 (-53.777, -54.256) -> (-53.8058, -54.2988)
  line L934 (-53.8058, -54.2988) -> (-53.8727, -54.3388)
  line L935 (-53.8727, -54.3388) -> (-53.949, -54.3631)
  line L936 (-53.949, -54.3631) -> (-54.0056, -54.3588)
  line L937 (-54.0056, -54.3588) -> (-54.0751, -54.2713)
  line L938 (-54.0751, -54.2713) -> (-54.1499, -54.1159)
  line L939 (-54.1499, -54.1159) -> (-54.2098, -53.942)
  line L940 (-54.2098, -53.942) -> (-54.2342, -53.7988)
  line L941 (-54.2342, -53.7988) -> (-54.2015, -53.6445)
  line L942 (-54.2015, -53.6445) -> (-54.1156, -53.4363)
  line L943 (-54.1156, -53.4363) -> (-53.9947, -53.2131)
  line L944 (-53.9947, -53.2131) -> (-53.857, -53.0139)
  line L945 (-53.857, -53.0139) -> (-53.7799, -52.892)
  line L946 (-53.7799, -52.892) -> (-53.7692, -52.8489)
  line L947 (-53.7692, -52.8489) -> (-53.777, -52.8158)
  line L948 (-53.777, -52.8158) -> (-53.8418, -52.6363)
  line L949 (-53.8418, -52.6363) -> (-53.9066, -52.3633)
  line L950 (-53.9066, -52.3633) -> (-53.957, -52.0689)
  line L951 (-53.957, -52.0689) -> (-53.9789, -51.8252)
  line L952 (-53.9789, -51.8252) -> (-53.9673, -51.5966)
  line L953 (-53.9673, -51.5966) -> (-53.9228, -51.4142)
  line L954 (-53.9228, -51.4142) -> (-53.8396, -51.261)
  line L955 (-53.8396, -51.261) -> (-53.7122, -51.1203)
  line L956 (-53.7122, -51.1203) -> (-53.6053, -51.0308)
  line L957 (-53.6053, -51.0308) -> (-53.5313, -50.9955)
  line L958 (-53.5313, -50.9955) -> (-53.4744, -51.0132)
  line L959 (-53.4744, -51.0132) -> (-53.4189, -51.0822)
  line L960 (-53.4189, -51.0822) -> (-53.3878, -51.1356)
  line L961 (-53.3878, -51.1356) -> (-53.3846, -51.1746)
  line L962 (-53.3846, -51.1746) -> (-53.4157, -51.2151)
  line L963 (-53.4157, -51.2151) -> (-53.4875, -51.2727)
  line L964 (-66.7284, 15.2692) -> (-69.8448, 15.2692)
  line L965 (-69.8448, 15.2692) -> (-69.8448, 11.3651)
  line L966 (-69.8448, 11.3651) -> (-71.4886, 12.1413)
  line L967 (-71.4886, 12.1413) -> (-71.4886, 16.9929)
  line L968 (-71.4886, 16.9929) -> (-63.5891, 16.9929)
  line L969 (-63.5891, 16.9929) -> (-63.0069, 17.6436)
  line L970 (-63.0069, 17.6436) -> (-61.7398, 16.4221)
  line L971 (-61.7398, 16.4221) -> (-62.7558, 15.2692)
  line L972 (-62.7558, 15.2692) -> (-62.0137, 14.9267)
  line L973 (-62.0137, 14.9267) -> (-62.0137, 11.3651)
  line L974 (-62.0137, 11.3651) -> (-63.6576, 12.1413)
  line L975 (-63.6576, 12.1413) -> (-63.6576, 15.2692)
  line L976 (-63.6576, 15.2692) -> (-66.4772, 15.2692)
  line L977 (-66.4772, 15.2692) -> (-65.2101, 14.687)
  line L978 (-65.2101, 14.687) -> (-65.2101, 11.6733)
  line L979 (-65.2101, 11.6733) -> (-66.7284, 12.381)
  line L980 (-66.7284, 12.381) -> (-66.7284, 15.2692)
  spline S0 degree 2 poles (-62.0137, 4.1847) (-63.3722, 2.8605) (-65.3014, 2.8605) knots 0 0 0 1 1 1
  spline S1 degree 2 poles (-65.3014, 2.8605) (-66.3402, 2.8605) (-68.4293, 3.6482) (-69.274, 4.3103) knots 0 0 0 1 2 2 2
  line L981 (-69.274, 4.3103) -> (-71.7512, 6.2623)
  line L982 (-71.7512, 6.2623) -> (-71.4886, 6.6505)
  line L983 (-71.4886, 6.6505) -> (-71.4886, 8.0888)
  line L984 (-71.4886, 8.0888) -> (-63.5891, 9.9952)
  line L985 (-63.5891, 9.9952) -> (-63.0069, 10.6459)
  line L986 (-63.0069, 10.6459) -> (-61.7398, 9.4244)
  line L987 (-61.7398, 9.4244) -> (-62.6302, 8.4199)
  line L988 (-62.6302, 8.4199) -> (-69.8448, 6.6961)
  line L989 (-69.8448, 6.6961) -> (-69.8448, 5.4861)
  line L990 (-69.8448, 5.4861) -> (-69.7192, 5.3947)
  spline S2 degree 2 poles (-69.7192, 5.3947) (-69.0115, 4.8696) (-67.3106, 4.2418) (-66.4201, 4.2418) knots 0 0 0 1 2 2 2
  spline S3 degree 2 poles (-66.4201, 4.2418) (-64.8905, 4.2418) (-63.6576, 5.2578) knots 0 0 0 1 1 1
  line L991 (-63.6576, 5.2578) -> (-63.6576, 7.0386)
  line L992 (-63.6576, 7.0386) -> (-62.0137, 6.2623)
  line L993 (-62.0137, 6.2623) -> (-62.0137, 4.1847)
  spline S4 degree 2 poles (-69.0571, -4.4454) (-69.6279, -4.4454) (-70.1758, -4.7651) (-70.4727, -5.1075) knots 0 0 0 1 2 2 2
  line L994 (-70.4727, -5.1075) -> (-71.7398, -3.8861)
  spline S5 degree 2 poles (-71.7398, -3.8861) (-71.7055, -3.8404) (-71.1462, -3.1783) (-70.1416, -2.7331) (-69.5252, -2.7331) knots 0 0 0 1 2 3 3 3
  line L995 (-69.5252, -2.7331) -> (-66.7284, -2.7331)
  line L996 (-66.7284, -2.7331) -> (-66.7284, -0.2445)
  line L997 (-66.7284, -0.2445) -> (-71.4886, -0.2445)
  line L998 (-71.4886, -0.2445) -> (-71.4886, 1.4792)
  line L999 (-71.4886, 1.4792) -> (-63.5891, 1.4792)
  line L1000 (-63.5891, 1.4792) -> (-63.0069, 2.1299)
  line L1001 (-63.0069, 2.1299) -> (-61.7398, 0.9084)
  line L1002 (-61.7398, 0.9084) -> (-62.7558, -0.2445)
  line L1003 (-62.7558, -0.2445) -> (-61.7398, -0.9066)
  spline S6 degree 2 poles (-61.7398, -0.9066) (-61.7398, -1.6715) (-62.4704, -3.3153) (-63.9316, -4.4454) (-64.9704, -4.4454) knots 0 0 0 1 2 3 3 3
  line L1004 (-64.9704, -4.4454) -> (-69.0571, -4.4454)
  line L1005 (-65.2101, -2.7331) -> (-65.1644, -2.7331)
  spline S7 degree 2 poles (-65.1644, -2.7331) (-64.3083, -2.7331) (-63.4749, -1.2491) (-63.4064, -0.2445) knots 0 0 0 1 2 2 2
  line L1006 (-63.4064, -0.2445) -> (-66.4201, -0.2445)
  line L1007 (-66.4201, -0.2445) -> (-65.2101, -0.8039)
  line L1008 (-65.2101, -0.8039) -> (-65.2101, -2.7331)
  line L1009 (-62.0137, -12.95) -> (-63.3037, -12.3564)
  line L1010 (-63.3037, -12.3564) -> (-71.7398, -12.3564)
  line L1011 (-71.7398, -12.3564) -> (-64.7078, -7.0938)
  line L1012 (-64.7078, -7.0938) -> (-69.8448, -7.0938)
  line L1013 (-69.8448, -7.0938) -> (-69.8448, -9.4911)
  line L1014 (-69.8448, -9.4911) -> (-71.4886, -8.7263)
  line L1015 (-71.4886, -8.7263) -> (-71.4886, -5.8381)
  line L1016 (-71.4886, -5.8381) -> (-70.0731, -6.4888)
  line L1017 (-70.0731, -6.4888) -> (-63.8973, -6.4888)
  line L1018 (-63.8973, -6.4888) -> (-63.0069, -5.8381)
  line L1019 (-63.0069, -5.8381) -> (-61.7398, -7.0596)
  line L1020 (-61.7398, -7.0596) -> (-68.0297, -11.7514)
  line L1021 (-68.0297, -11.7514) -> (-63.6576, -11.7514)
  line L1022 (-63.6576, -11.7514) -> (-63.6576, -9.7993)
  line L1023 (-63.6576, -9.7993) -> (-62.0137, -10.5642)
  line L1024 (-62.0137, -10.5642) -> (-62.0137, -12.95)
  spline S8 degree 2 poles (-64.8334, -19.5368) (-64.8334, -20.5756) (-65.8494, -21.7514) (-66.6941, -21.7514) knots 0 0 0 1 2 2 2
  spline S9 degree 2 poles (-66.6941, -21.7514) (-67.2306, -21.7514) (-68.4064, -21.2833) (-69.0115, -20.7925) knots 0 0 0 1 2 2 2
  line L1025 (-69.0115, -20.7925) -> (-71.7512, -18.6349)
  line L1026 (-71.7512, -18.6349) -> (-71.4544, -18.1441)
  spline S10 degree 2 poles (-71.4544, -18.1441) (-71.3288, -16.7742) (-70.0389, -14.7537) (-67.9612, -13.6806) (-66.6484, -13.6806) knots 0 0 0 1 2 3 3 3
  spline S11 degree 2 poles (-66.6484, -13.6806) (-66.0206, -13.6806) (-64.7877, -14.1372) (-63.7147, -14.7993) (-62.9042, -15.3815) knots 0 0 0 1 2 3 3 3
  spline S12 degree 2 poles (-62.9042, -15.3815) (-62.2535, -15.861) (-61.7398, -16.1806) knots 0 0 0 1 1 1
  line L1027 (-61.7398, -16.1806) -> (-62.0137, -16.5801)
  line L1028 (-62.0137, -16.5801) -> (-62.0137, -20.4386)
  line L1029 (-62.0137, -20.4386) -> (-63.6576, -19.6737)
  line L1030 (-63.6576, -19.6737) -> (-63.6576, -15.5642)
  spline S13 degree 2 poles (-63.6576, -15.5642) (-64.1713, -15.2902) (-65.0389, -15.0276) (-65.564, -15.0276) knots 0 0 0 1 2 2 2
  spline S14 degree 2 poles (-65.564, -15.0276) (-67.6416, -15.0276) (-69.7192, -17.3336) (-69.8334, -19.4112) knots 0 0 0 1 2 2 2
  line L1031 (-69.8334, -19.4112) -> (-69.4567, -19.7194)
  spline S15 degree 2 poles (-69.4567, -19.7194) (-68.9316, -20.1304) (-67.9727, -20.5413) (-67.5845, -20.5413) knots 0 0 0 1 2 2 2
  spline S16 degree 2 poles (-67.5845, -20.5413) (-67.0023, -20.5413) (-66.3402, -19.7194) (-66.3402, -18.9546) knots 0 0 0 1 2 2 2
  line L1032 (-66.3402, -18.9546) -> (-66.3402, -16.1692)
  line L1033 (-66.3402, -16.1692) -> (-64.8334, -16.8769)
  line L1034 (-64.8334, -16.8769) -> (-64.8334, -19.5368)
  line L1035 (-66.7284, -24.845) -> (-69.8448, -24.845)
  line L1036 (-69.8448, -24.845) -> (-69.8448, -28.7491)
  line L1037 (-69.8448, -28.7491) -> (-71.4886, -27.9728)
  line L1038 (-71.4886, -27.9728) -> (-71.4886, -23.1212)
  line L1039 (-71.4886, -23.1212) -> (-63.5891, -23.1212)
  line L1040 (-63.5891, -23.1212) -> (-63.0069, -22.4705)
  line L1041 (-63.0069, -22.4705) -> (-61.7398, -23.692)
  line L1042 (-61.7398, -23.692) -> (-62.7558, -24.845)
  line L1043 (-62.7558, -24.845) -> (-62.0137, -25.1874)
  line L1044 (-62.0137, -25.1874) -> (-62.0137, -28.7491)
  line L1045 (-62.0137, -28.7491) -> (-63.6576, -27.9728)
  line L1046 (-63.6576, -27.9728) -> (-63.6576, -24.845)
  line L1047 (-63.6576, -24.845) -> (-66.4772, -24.845)
  line L1048 (-66.4772, -24.845) -> (-65.2101, -25.4272)
  line L1049 (-65.2101, -25.4272) -> (-65.2101, -28.4409)
  line L1050 (-65.2101, -28.4409) -> (-66.7284, -27.7331)
  line L1051 (-66.7284, -27.7331) -> (-66.7284, -24.845)
  line L1052 (-69.8448, -32.0253) -> (-69.8448, -35.9409)
  line L1053 (-69.8448, -35.9409) -> (-71.4886, -35.1646)
  line L1054 (-71.4886, -35.1646) -> (-71.4886, -30.3016)
  line L1055 (-71.4886, -30.3016) -> (-63.6576, -30.3016)
  line L1056 (-63.6576, -30.3016) -> (-63.6576, -29.4683)
  line L1057 (-63.6576, -29.4683) -> (-62.0137, -30.2331)
  line L1058 (-62.0137, -30.2331) -> (-62.0137, -32.619)
  line L1059 (-62.0137, -32.619) -> (-63.3037, -32.0253)
  line L1060 (-63.3037, -32.0253) -> (-69.8448, -32.0253)
  line L1061 (-62.0137, -39.8107) -> (-63.3037, -39.2171)
  line L1062 (-63.3037, -39.2171) -> (-71.4886, -39.2171)
  line L1063 (-71.4886, -39.2171) -> (-71.4886, -37.4934)
  line L1064 (-71.4886, -37.4934) -> (-63.6576, -37.4934)
  line L1065 (-63.6576, -37.4934) -> (-63.6576, -36.66)
  line L1066 (-63.6576, -36.66) -> (-62.0137, -37.4249)
  line L1067 (-62.0137, -37.4249) -> (-62.0137, -39.8107)
  spline S17 degree 2 poles (-66.58, -48.2126) (-67.2192, -48.2126) (-68.532, -47.6989) (-69.6964, -46.9569) (-70.5754, -46.3404) knots 0 0 0 1 2 3 3 3
  spline S18 degree 2 poles (-70.5754, -46.3404) (-70.7923, -46.192) (-71.5, -45.7011) (-71.7512, -45.5299) knots 0 0 0 1 2 2 2
  line L1068 (-71.7512, -45.5299) -> (-71.4658, -45.1418)
  spline S19 degree 2 poles (-71.4658, -45.1418) (-71.3631, -43.7263) (-70.0845, -41.6486) (-67.9841, -40.5413) (-66.6484, -40.5413) knots 0 0 0 1 2 3 3 3
  spline S20 degree 2 poles (-66.6484, -40.5413) (-66.0206, -40.5413) (-64.7877, -40.9979) (-63.7147, -41.66) (-62.9042, -42.2422) knots 0 0 0 1 2 3 3 3
  spline S21 degree 2 poles (-62.9042, -42.2422) (-62.2535, -42.7217) (-61.7398, -43.0413) knots 0 0 0 1 1 1
  line L1069 (-61.7398, -43.0413) -> (-62.0137, -43.4409)
  line L1070 (-62.0137, -43.4409) -> (-62.0137, -46.1007)
  line L1071 (-62.0137, -46.1007) -> (-62.3905, -45.918)
  spline S22 degree 2 poles (-62.3905, -45.918) (-63.0069, -47.0025) (-65.1873, -48.2126) (-66.58, -48.2126) knots 0 0 0 1 2 2 2
  spline S23 degree 2 poles (-65.564, -41.8884) (-67.6188, -41.8884) (-69.7078, -44.1372) (-69.8334, -46.1806) knots 0 0 0 1 2 2 2
  spline S24 degree 2 poles (-69.8334, -46.1806) (-69.2055, -46.5573) (-68.201, -46.9112) (-67.6758, -46.9112) knots 0 0 0 1 2 2 2
  spline S25 degree 2 poles (-67.6758, -46.9112) (-66.0434, -46.9112) (-64.0457, -45.4728) (-63.6576, -44.1829) knots 0 0 0 1 2 2 2
  line L1072 (-63.6576, -44.1829) -> (-63.6576, -42.4249)
  spline S26 degree 2 poles (-63.6576, -42.4249) (-64.1713, -42.1509) (-65.0389, -41.8884) (-65.564, -41.8884) knots 0 0 0 1 2 2 2
  line L1073 (-62.0137, -56.0436) -> (-63.3037, -55.45)
  line L1074 (-63.3037, -55.45) -> (-71.7398, -55.45)
  line L1075 (-71.7398, -55.45) -> (-64.7078, -50.1874)
  line L1076 (-64.7078, -50.1874) -> (-69.8448, -50.1874)
  line L1077 (-69.8448, -50.1874) -> (-69.8448, -52.5847)
  line L1078 (-69.8448, -52.5847) -> (-71.4886, -51.8199)
  line L1079 (-71.4886, -51.8199) -> (-71.4886, -48.9317)
  line L1080 (-71.4886, -48.9317) -> (-70.0731, -49.5824)
  line L1081 (-70.0731, -49.5824) -> (-63.8973, -49.5824)
  line L1082 (-63.8973, -49.5824) -> (-63.0069, -48.9317)
  line L1083 (-63.0069, -48.9317) -> (-61.7398, -50.1532)
  line L1084 (-61.7398, -50.1532) -> (-68.0297, -54.845)
  line L1085 (-68.0297, -54.845) -> (-63.6576, -54.845)
  line L1086 (-63.6576, -54.845) -> (-63.6576, -52.8929)
  line L1087 (-63.6576, -52.8929) -> (-62.0137, -53.6578)
  line L1088 (-62.0137, -53.6578) -> (-62.0137, -56.0436)
  line L1089 (-74.3267, -17.9742) -> (-75.4141, -17.2042)
  line L1090 (-75.4141, -17.2042) -> (-75.4141, -15.2418)
  line L1091 (-75.4141, -15.2418) -> (-76.8854, -15.2418)
  line L1092 (-76.8854, -15.2418) -> (-76.3622, -14.2914)
  line L1093 (-76.3622, -14.2914) -> (-73.3854, -14.2914)
  line L1094 (-73.3854, -14.2914) -> (-73.3854, -17.3093)
  line L1095 (-73.3854, -17.3093) -> (-74.3267, -17.9742)
  line L1096 (-74.3861, -16.9986) -> (-74.1279, -16.7976)
  line L1097 (-74.1279, -16.7976) -> (-74.1279, -15.2418)
  line L1098 (-74.1279, -15.2418) -> (-74.6556, -15.2418)
  line L1099 (-74.6556, -15.2418) -> (-74.6556, -16.7976)
  line L1100 (-74.6556, -16.7976) -> (-74.3861, -16.9986)
  line L1101 (-75.6403, -21.5975) -> (-76.3874, -20.9373)
  line L1102 (-76.3874, -20.9373) -> (-76.3874, -18.23)
  line L1103 (-76.3874, -18.23) -> (-73.4082, -18.23)
  line L1104 (-73.4082, -18.23) -> (-72.8782, -19.1804)
  line L1105 (-72.8782, -19.1804) -> (-75.6403, -19.1804)
  line L1106 (-75.6403, -19.1804) -> (-75.6403, -21.5975)
  line L1107 (-75.6928, -25.1752) -> (-76.3828, -24.5058)
  line L1108 (-76.3828, -24.5058) -> (-76.3828, -22.3309)
  line L1109 (-76.3828, -22.3309) -> (-75.6928, -21.6615)
  line L1110 (-75.6928, -21.6615) -> (-73.3785, -21.6615)
  line L1111 (-73.3785, -21.6615) -> (-73.3854, -22.6119)
  line L1112 (-73.3854, -22.6119) -> (-75.6403, -22.6119)
  line L1113 (-75.6403, -22.6119) -> (-75.6403, -24.2202)
  line L1114 (-75.6403, -24.2202) -> (-73.4082, -24.2202)
  line L1115 (-73.4082, -24.2202) -> (-72.8782, -25.1752)
  line L1116 (-72.8782, -25.1752) -> (-75.6928, -25.1752)
  line L1117 (-75.4438, -29.6302) -> (-76.3828, -28.9653)
  line L1118 (-76.3828, -28.9653) -> (-76.3828, -25.623)
  line L1119 (-76.3828, -25.623) -> (-75.6403, -26.2764)
  line L1120 (-75.6403, -26.2764) -> (-75.6403, -28.417)
  line L1121 (-75.6403, -28.417) -> (-75.4415, -28.593)
  line L1122 (-75.4415, -28.593) -> (-75.2314, -28.417)
  line L1123 (-75.2314, -28.417) -> (-75.2314, -26.2672)
  line L1124 (-75.2314, -26.2672) -> (-74.3267, -25.623)
  line L1125 (-74.3267, -25.623) -> (-73.3854, -26.2878)
  line L1126 (-73.3854, -26.2878) -> (-73.3854, -29.6302)
  line L1127 (-73.3854, -29.6302) -> (-74.1279, -28.9699)
  line L1128 (-74.1279, -28.9699) -> (-74.1279, -26.8338)
  line L1129 (-74.1279, -26.8338) -> (-74.3267, -26.6556)
  line L1130 (-74.3267, -26.6556) -> (-74.5368, -26.8338)
  line L1131 (-74.5368, -26.8338) -> (-74.5368, -28.9836)
  line L1132 (-74.5368, -28.9836) -> (-75.4438, -29.6302)
  line L1133 (-75.6928, -33.4843) -> (-76.3828, -32.8149)
  line L1134 (-76.3828, -32.8149) -> (-76.3828, -30.6399)
  line L1135 (-76.3828, -30.6399) -> (-75.6928, -29.9706)
  line L1136 (-75.6928, -29.9706) -> (-73.3785, -29.9706)
  line L1137 (-73.3785, -29.9706) -> (-73.3854, -30.921)
  line L1138 (-73.3854, -30.921) -> (-75.6403, -30.921)
  line L1139 (-75.6403, -30.921) -> (-75.6403, -32.5293)
  line L1140 (-75.6403, -32.5293) -> (-73.4082, -32.5293)
  line L1141 (-73.4082, -32.5293) -> (-72.8782, -33.4843)
  line L1142 (-72.8782, -33.4843) -> (-75.6928, -33.4843)
  line L1143 (-74.3267, -40.1553) -> (-75.4141, -39.3854)
  line L1144 (-75.4141, -39.3854) -> (-75.4141, -37.4229)
  line L1145 (-75.4141, -37.4229) -> (-76.8854, -37.4229)
  line L1146 (-76.8854, -37.4229) -> (-76.3622, -36.4725)
  line L1147 (-76.3622, -36.4725) -> (-73.3854, -36.4725)
  line L1148 (-73.3854, -36.4725) -> (-73.3854, -39.4905)
  line L1149 (-73.3854, -39.4905) -> (-74.3267, -40.1553)
  line L1150 (-74.3861, -39.1798) -> (-74.1279, -38.9787)
  line L1151 (-74.1279, -38.9787) -> (-74.1279, -37.4229)
  line L1152 (-74.1279, -37.4229) -> (-74.6556, -37.4229)
  line L1153 (-74.6556, -37.4229) -> (-74.6556, -38.9787)
  line L1154 (-74.6556, -38.9787) -> (-74.3861, -39.1798)
  line L1155 (-75.6403, -43.7787) -> (-76.3874, -43.1184)
  line L1156 (-76.3874, -43.1184) -> (-76.3874, -40.4112)
  line L1157 (-76.3874, -40.4112) -> (-73.4082, -40.4112)
  line L1158 (-73.4082, -40.4112) -> (-72.8782, -41.3616)
  line L1159 (-72.8782, -41.3616) -> (-75.6403, -41.3616)
  line L1160 (-75.6403, -41.3616) -> (-75.6403, -43.7787)
  line L1161 (-75.6928, -47.3563) -> (-76.3828, -46.6869)
  line L1162 (-76.3828, -46.6869) -> (-76.3828, -44.512)
  line L1163 (-76.3828, -44.512) -> (-75.6928, -43.8426)
  line L1164 (-75.6928, -43.8426) -> (-73.3785, -43.8426)
  line L1165 (-73.3785, -43.8426) -> (-73.3854, -44.793)
  line L1166 (-73.3854, -44.793) -> (-75.6403, -44.793)
  line L1167 (-75.6403, -44.793) -> (-75.6403, -46.4014)
  line L1168 (-75.6403, -46.4014) -> (-73.4082, -46.4014)
  line L1169 (-73.4082, -46.4014) -> (-72.8782, -47.3563)
  line L1170 (-72.8782, -47.3563) -> (-75.6928, -47.3563)
  line L1171 (-75.4438, -51.8113) -> (-76.3828, -51.1465)
  line L1172 (-76.3828, -51.1465) -> (-76.3828, -47.8041)
  line L1173 (-76.3828, -47.8041) -> (-75.6403, -48.4575)
  line L1174 (-75.6403, -48.4575) -> (-75.6403, -50.5982)
  line L1175 (-75.6403, -50.5982) -> (-75.4415, -50.7741)
  line L1176 (-75.4415, -50.7741) -> (-75.2314, -50.5982)
  line L1177 (-75.2314, -50.5982) -> (-75.2314, -48.4484)
  line L1178 (-75.2314, -48.4484) -> (-74.3267, -47.8041)
  line L1179 (-74.3267, -47.8041) -> (-73.3854, -48.4689)
  line L1180 (-73.3854, -48.4689) -> (-73.3854, -51.8113)
  line L1181 (-73.3854, -51.8113) -> (-74.1279, -51.151)
  line L1182 (-74.1279, -51.151) -> (-74.1279, -49.0149)
  line L1183 (-74.1279, -49.0149) -> (-74.3267, -48.8367)
  line L1184 (-74.3267, -48.8367) -> (-74.5368, -49.0149)
  line L1185 (-74.5368, -49.0149) -> (-74.5368, -51.1648)
  line L1186 (-74.5368, -51.1648) -> (-75.4438, -51.8113)
  line L1187 (-75.6928, -55.6654) -> (-76.3828, -54.996)
  line L1188 (-76.3828, -54.996) -> (-76.3828, -52.8211)
  line L1189 (-76.3828, -52.8211) -> (-75.6928, -52.1517)
  line L1190 (-75.6928, -52.1517) -> (-73.3785, -52.1517)